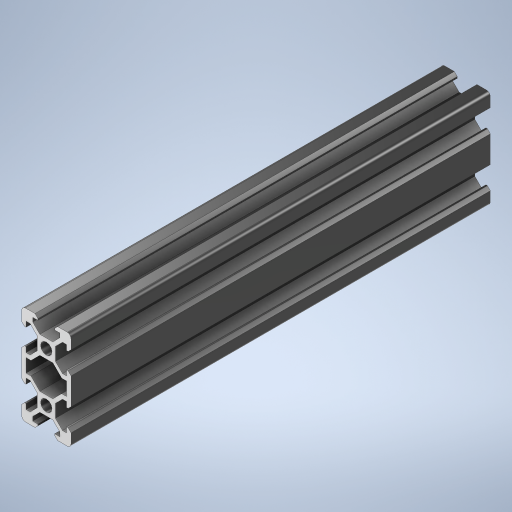
# Autodesk Inventor part: 2040aluminum_extrusion_black
Saved by Autodesk Inventor 2024.2 (Build 282272000, 272)
## iProperties
Created: 2021-10-28
Part Number: 2040aluminum_extrusion_black
Material: Aluminum 6061
Document SubType Name: Modeling
Designer: casper
Density: 2.7 g/cm^3
Appearance: Satin - Black
Author: casper
Autodesk Inventor part; units mm, degrees
ref_plane "YZ Plane" through (0, 0, 0) normal (1, 0, 0) x (0, 1, 0)
ref_plane "XZ Plane" through (0, 0, 0) normal (0, 1, 0) x (-1, 0, 0)
ref_plane "XY Plane" through (0, 0, 0) normal (0, 0, 1) x (1, 0, 0)
sketch "Sketch1" plane through (0, 0, 0) normal (0, 0, 1) x (1, 0, 0)
  line L0 (0, 3.7) -> (-2.6393, 3.7)
  line L1 (-2.6393, 3.7) -> (-5.5, 6.5607)
  line L2 (-5.5, 6.5607) -> (-5.5, 8.2)
  line L3 (-5.5, 8.2) -> (-3.395, 8.2)
  line L4 (-3.395, 8.2) -> (-3.395, 10)
  line L5 (-3.395, 10) -> (-10, 10)
  line L6 (-10, 10) -> (-10, 3.395)
  line L7 (-10, 3.395) -> (-8.2, 3.395)
  line L8 (-8.2, 3.395) -> (-8.2, 5.5)
  line L9 (-8.2, 5.5) -> (-6.5607, 5.5)
  line L10 (-6.5607, 5.5) -> (-3.7, 2.6393)
  line L11 (-3.7, 2.6393) -> (-3.7, 0)
  line L12 (0, 0) -> (-10, 10) construction
  circle A0 centre (0, 0) radius 2.3
  line L13 (-22.6601, 0) -> (65.9605, 0) projected
  line L14 (-3.7, 0) -> (0, 0)
  line L15 (0, 0) -> (0, 3.7)
  line L16 (11.2521, 18.9743) -> (53.3004, 18.9743) construction
  line L17 (53.3004, 18.9743) -> (53.3004, -5.624) construction
  line L18 (53.3004, -5.624) -> (11.2521, -5.624) construction
  line L19 (11.2521, -5.624) -> (11.2521, 18.9743) construction
  point P0 (-2.3, 0)
  point P1 (0, 2.3)
  dimension "d0" = 1.5
  dimension "d6" = 6.3
  dimension "d9" = 4.6
  dimension "d18" = 135
  dimension "d22" = 20
  dimension "d34" = 11
  dimension "d35" = 6.79
  dimension "d36" = 1.8
  constraints: 30 end point, 6 equal length, 6 perpendicular, 2 horizontal, 2 parallel, 2 vertical, 1 centre point, 1 coincident, 2 other
  measures "d0" distance between parallel lines of L1 L10
  measures "d6" distance between parallel lines of L0 L5
  measures "d9" diameter of A0
  measures "d18" angle of L13 L12
  measures "d22" diameter of L5 L14
  measures "d34" diameter of L2 L15
  measures "d35" diameter of L4 L15
  measures "d36" distance between parallel lines of L5 L3
extrude "Extrusion1" add sketch "Sketch1" along normal mid plane 170 contours L15 A0 L13 L11 L10 L9 L8 L7 L6 L5 L4 L3 L2 L1 L0
pattern_circular "Circular Pattern1" count 4 over 360 about axis through (0, 0, -10) along (0, 0, 1) of "Extrusion1"
chamfer "Chamfer1" distance 1.185 angle 45 8 edges at (-3.395, 10, 0) (3.395, 10, 0) (10, 3.395, 0) (10, -3.395, 0) (3.395, -10, 0) (-3.395, -10, 0) (-10, -3.395, 0) (-10, 3.395, 0)
ref_plane "Work Plane1" through (4.58, 10, 85) normal (0, 1, 0) x (1, 0, 0)
mirror "Mirror1" about plane through (4.58, 10, 85) normal (0, 1, 0)
sketch "Sketch2" plane through (0, 0, 85) normal (0, 0, 1) x (1, 0, 0)
  line L0 (-10, 4.58) -> (-10, 15.42) projected
  line L1 (-8.815, 3.395) -> (-10, 4.58) projected
  line L2 (-8.815, 3.395) -> (-8.2, 3.395) projected
  line L3 (-8.2, 3.395) -> (-8.2, 5.5) projected
  line L4 (-8.2, 5.5) -> (-6.5607, 5.5) projected
  line L5 (-6.5607, 5.5) -> (-3.7, 2.6393) projected
  line L6 (-3.7, -2.6393) -> (-6.5607, -5.5) projected
  line L7 (-6.5607, -5.5) -> (-8.2, -5.5) projected
  line L8 (-8.2, -5.5) -> (-8.2, -3.395) projected
  line L9 (-8.2, -3.395) -> (-8.815, -3.395) projected
  line L10 (-10, -4.58) -> (-8.815, -3.395) projected
  line L11 (-10, -4.58) -> (-10, -10) projected
  line L12 (-10, -10) -> (-4.58, -10) projected
  line L13 (-3.395, -8.815) -> (-4.58, -10) projected
  line L14 (-3.395, -8.815) -> (-3.395, -8.2) projected
  line L15 (-3.395, -8.2) -> (-5.5, -8.2) projected
  line L16 (-5.5, -8.2) -> (-5.5, -6.5607) projected
  line L17 (-5.5, -6.5607) -> (-2.6393, -3.7) projected
  line L18 (2.6393, -3.7) -> (5.5, -6.5607) projected
  line L19 (5.5, -6.5607) -> (5.5, -8.2) projected
  line L20 (5.5, -8.2) -> (3.395, -8.2) projected
  line L21 (3.395, -8.2) -> (3.395, -8.815) projected
  line L22 (4.58, -10) -> (3.395, -8.815) projected
  line L23 (4.58, -10) -> (10, -10) projected
  line L24 (10, -10) -> (10, -4.58) projected
  line L25 (8.815, -3.395) -> (10, -4.58) projected
  line L26 (8.815, -3.395) -> (8.2, -3.395) projected
  line L27 (8.2, -3.395) -> (8.2, -5.5) projected
  line L28 (8.2, -5.5) -> (6.5607, -5.5) projected
  line L29 (6.5607, -5.5) -> (3.7, -2.6393) projected
  line L30 (3.7, 2.6393) -> (6.5607, 5.5) projected
  line L31 (6.5607, 5.5) -> (8.2, 5.5) projected
  line L32 (8.2, 5.5) -> (8.2, 3.395) projected
  line L33 (8.2, 3.395) -> (8.815, 3.395) projected
  line L34 (10, 4.58) -> (8.815, 3.395) projected
  line L35 (10, 4.58) -> (10, 15.42) projected
  line L36 (10, 15.42) -> (8.815, 16.605) projected
  line L37 (8.2, 16.605) -> (8.815, 16.605) projected
  line L38 (8.2, 14.5) -> (8.2, 16.605) projected
  line L39 (6.5607, 14.5) -> (8.2, 14.5) projected
  line L40 (3.7, 17.3607) -> (6.5607, 14.5) projected
  line L41 (6.5607, 25.5) -> (3.7, 22.6393) projected
  line L42 (8.2, 25.5) -> (6.5607, 25.5) projected
  line L43 (8.2, 23.395) -> (8.2, 25.5) projected
  line L44 (8.815, 23.395) -> (8.2, 23.395) projected
  line L45 (8.815, 23.395) -> (10, 24.58) projected
  line L46 (10, 30) -> (10, 24.58) projected
  line L47 (4.58, 30) -> (10, 30) projected
  line L48 (4.58, 30) -> (3.395, 28.815) projected
  line L49 (3.395, 28.2) -> (3.395, 28.815) projected
  line L50 (5.5, 28.2) -> (3.395, 28.2) projected
  line L51 (5.5, 26.5607) -> (5.5, 28.2) projected
  line L52 (2.6393, 23.7) -> (5.5, 26.5607) projected
  line L53 (-5.5, 26.5607) -> (-2.6393, 23.7) projected
  line L54 (-5.5, 28.2) -> (-5.5, 26.5607) projected
  line L55 (-3.395, 28.2) -> (-5.5, 28.2) projected
  line L56 (-3.395, 28.815) -> (-3.395, 28.2) projected
  line L57 (-3.395, 28.815) -> (-4.58, 30) projected
  line L58 (-10, 30) -> (-4.58, 30) projected
  line L59 (-10, 24.58) -> (-10, 30) projected
  line L60 (-10, 24.58) -> (-8.815, 23.395) projected
  line L61 (-8.2, 23.395) -> (-8.815, 23.395) projected
  line L62 (-8.2, 25.5) -> (-8.2, 23.395) projected
  line L63 (-6.5607, 25.5) -> (-8.2, 25.5) projected
  line L64 (-3.7, 22.6393) -> (-6.5607, 25.5) projected
  line L65 (-6.5607, 14.5) -> (-3.7, 17.3607) projected
  line L66 (-8.2, 14.5) -> (-6.5607, 14.5) projected
  line L67 (-8.2, 16.605) -> (-8.2, 14.5) projected
  line L68 (-8.815, 16.605) -> (-8.2, 16.605) projected
  line L69 (-8.815, 16.605) -> (-10, 15.42) projected
  circle A0 centre (0, 20) radius 2.3 projected
  line L70 (-4.58, 10) -> (-3.395, 11.185) projected
  line L71 (-3.395, 11.8) -> (-3.395, 11.185) projected
  line L72 (-5.5, 11.8) -> (-3.395, 11.8) projected
  line L73 (-5.5, 13.4393) -> (-5.5, 11.8) projected
  line L74 (-2.6393, 16.3) -> (-5.5, 13.4393) projected
  line L75 (5.5, 13.4393) -> (2.6393, 16.3) projected
  line L76 (5.5, 11.8) -> (5.5, 13.4393) projected
  line L77 (3.395, 11.8) -> (5.5, 11.8) projected
  line L78 (3.395, 11.185) -> (3.395, 11.8) projected
  line L79 (3.395, 11.185) -> (4.58, 10) projected
  line L80 (3.395, 8.815) -> (4.58, 10) projected
  line L81 (3.395, 8.815) -> (3.395, 8.2) projected
  line L82 (3.395, 8.2) -> (5.5, 8.2) projected
  line L83 (5.5, 8.2) -> (5.5, 6.5607) projected
  line L84 (5.5, 6.5607) -> (2.6393, 3.7) projected
  line L85 (-2.6393, 3.7) -> (-5.5, 6.5607) projected
  line L86 (-5.5, 6.5607) -> (-5.5, 8.2) projected
  line L87 (-5.5, 8.2) -> (-3.395, 8.2) projected
  line L88 (-3.395, 8.2) -> (-3.395, 8.815) projected
  line L89 (-4.58, 10) -> (-3.395, 8.815) projected
  circle A1 centre (0, 0) radius 2.3 projected
  line L90 (-5.5, 8.2) -> (-5.5, 6.5607) projected
  line L91 (-5.5, 6.5607) -> (-6.2393, 7.3)
  line L92 (-5.5, 6.5607) -> (-2.6393, 3.7) projected
  line L93 (-6.2393, 7.3) -> (-8.2, 7.3)
  line L94 (-8.2, 7.3) -> (-8.2, 12.7)
  line L95 (-8.2, 12.7) -> (-6.2393, 12.7)
  line L96 (-6.2393, 12.7) -> (-5.5, 13.4393)
  line L97 (-2.6393, 16.3) -> (-5.5, 13.4393) projected
  line L98 (-8.2, 16.605) -> (-8.2, 14.5) projected
  line L99 (-3.7, 2.6393) -> (-3.7, -2.6393) projected
  line L100 (-2.6393, -3.7) -> (2.6393, -3.7) projected
  line L101 (3.7, -2.6393) -> (3.7, 2.6393) projected
  line L102 (3.7, 22.6393) -> (3.7, 17.3607) projected
  line L103 (-2.6393, 23.7) -> (2.6393, 23.7) projected
  line L104 (-3.7, 17.3607) -> (-3.7, 22.6393) projected
  line L105 (2.6393, 16.3) -> (-2.6393, 16.3) projected
  line L106 (2.6393, 3.7) -> (-2.6393, 3.7) projected
  dimension "d42" = 1.8
  constraints: 10 end point, 3 collinear, 2 perpendicular, 1 horizontal, 1 vertical alignment
  measures "d42" distance between parallel lines of L4 L93
extrude "Extrusion2" cut sketch "Sketch2" against normal through all contours L89 L88 L87 L86 L91 L93 L94 L95 L96 L73 L72 L71 L70
fillet "Fillet2" radius 1.5 4 edges at (-10, 30, 0) (10, 30, 0) (10, -10, 0) (-10, -10, 0)
mirror "Mirror2" about plane through (0, 0, 0) normal (1, 0, 0) of "Extrusion2"
body "Solid1"
